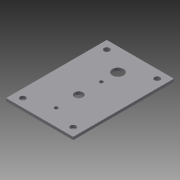
# Autodesk Inventor part: Gearbox plate
Saved by Autodesk Inventor 2015 (Build 190159000, 159)
## iProperties
Created: 2015-02-21
Part Number: Gearbox plate
Material: Generic
Document SubType Name: Modeling
Designer: szymsea16
Density: 1 g/cm^3
Appearance: Default
Author: szymsea16
Autodesk Inventor part; units mm, degrees
ref_plane "YZ Plane" through (0, 0, 0) normal (1, 0, 0) x (0, 1, 0)
ref_plane "XZ Plane" through (0, 0, 0) normal (0, 1, 0) x (-1, 0, 0)
ref_plane "XY Plane" through (0, 0, 0) normal (0, 0, 1) x (1, 0, 0)
sketch "Sketch1" plane through (0, 0, 0) normal (0, 1, 0) x (-1, 0, 0)
  line L0 (0, 0) -> (76.2, 0)
  line L1 (76.2, 0) -> (76.2, -114.3)
  line L2 (76.2, -114.3) -> (0, -114.3)
  line L3 (0, -114.3) -> (0, 0)
  dimension "d0" = 76.2
  dimension "d1" = 114.3
  constraints: 8 end point, 2 parallel, 1 horizontal, 1 perpendicular
  measures "d0" distance of L1.end L2.end
  measures "d1" distance of L0.end L1.end
extrude "Extrusion1" add sketch "Sketch1" along normal blind 3.175
hole "Hole1" at (-9.525, 3.175, -9.525) direction (0, -1, 0) diameter 6.35 depth 25.4 tip angle 118
hole "Hole2" at (-9.525, 3.175, -104.775) direction (0, -1, 0) diameter 6.35 depth 25.4 tip angle 118
hole "Hole3" at (-66.675, 3.175, -104.775) direction (0, -1, 0) diameter 6.35 depth 25.4 tip angle 118
hole "Hole4" at (-66.675, 3.175, -9.525) direction (0, -1, 0) diameter 6.35 depth 25.4 tip angle 118
hole "Hole5" at (-38.1, 3.175, -88.9) direction (0, -1, 0) diameter 12.7 depth 25.4 tip angle 118
hole "Hole6" at (-38.1, 3.175, -44.45) direction (0, -1, 0) diameter 9.525 depth 25.4 tip angle 118
hole "Hole7" at (-38.1, 3.175, -18.8468) direction (0, -1, 0) diameter 4.0386 depth 25.4 tip angle 118
hole "Hole8" at (-38.1, 3.175, -70.0532) direction (0, -1, 0) diameter 4.0386 depth 25.4 tip angle 118
body "Solid1"
